Autodesk Fusion 360 part; units mm, degrees
(part 13 of 14)
  arc A3739 (79.673, 23.2351) -> (79.673, 23.4129) centre (79.673, 23.324) ccw
  arc A3740 (71.673, 22.4351) -> (71.673, 22.6129) centre (71.673, 22.524) ccw
  arc A3741 (78.073, 23.4129) -> (78.073, 23.2351) centre (78.073, 23.324) ccw
  arc A3742 (73.273, 22.4351) -> (73.273, 22.6129) centre (73.273, 22.524) ccw
  arc A3743 (73.273, 22.4351) -> (73.273, 22.6129) centre (73.273, 22.524) ccw
  arc A3744 (78.073, 23.4129) -> (78.073, 23.2351) centre (78.073, 23.324) ccw
  arc A3745 (75.673, 23.4129) -> (75.673, 23.2351) centre (75.673, 23.324) ccw
  arc A3746 (74.873, 23.2351) -> (74.873, 23.4129) centre (74.873, 23.324) ccw
  arc A3747 (74.073, 23.4129) -> (74.073, 23.2351) centre (74.073, 23.324) ccw
  arc A3748 (74.073, 23.4129) -> (74.073, 23.2351) centre (74.073, 23.324) ccw
  arc A3749 (74.073, 23.2351) -> (74.073, 23.4129) centre (74.073, 23.324) ccw
  arc A3750 (78.873, 23.4129) -> (78.873, 23.2351) centre (78.873, 23.324) ccw
  arc A3751 (80.473, 23.4129) -> (80.473, 23.2351) centre (80.473, 23.324) ccw
  arc A3752 (78.073, 23.2351) -> (78.073, 23.4129) centre (78.073, 23.324) ccw
  arc A3753 (79.673, 23.4129) -> (79.673, 23.2351) centre (79.673, 23.324) ccw
  arc A3754 (76.473, 23.4129) -> (76.473, 23.2351) centre (76.473, 23.324) ccw
  arc A3755 (74.873, 23.4129) -> (74.873, 23.2351) centre (74.873, 23.324) ccw
  arc A3756 (72.473, 22.4351) -> (72.473, 22.6129) centre (72.473, 22.524) ccw
  arc A3757 (78.073, 23.2351) -> (78.073, 23.4129) centre (78.073, 23.324) ccw
  arc A3758 (76.473, 23.4129) -> (76.473, 23.2351) centre (76.473, 23.324) ccw
  arc A3759 (77.273, 23.4129) -> (77.273, 23.2351) centre (77.273, 23.324) ccw
  arc A3760 (76.473, 23.2351) -> (76.473, 23.4129) centre (76.473, 23.324) ccw
  arc A3761 (78.873, 23.4129) -> (78.873, 23.2351) centre (78.873, 23.324) ccw
  arc A3762 (72.473, 22.6129) -> (72.473, 22.4351) centre (72.473, 22.524) ccw
  arc A3763 (80.473, 23.2351) -> (80.473, 23.4129) centre (80.473, 23.324) ccw
  arc A3764 (71.673, 22.6129) -> (71.673, 22.4351) centre (71.673, 22.524) ccw
  arc A3765 (79.673, 23.2351) -> (79.673, 23.4129) centre (79.673, 23.324) ccw
  arc A3766 (78.873, 23.2351) -> (78.873, 23.4129) centre (78.873, 23.324) ccw
  arc A3767 (79.673, 23.2351) -> (79.673, 23.4129) centre (79.673, 23.324) ccw
  arc A3768 (73.273, 22.6129) -> (73.273, 22.4351) centre (73.273, 22.524) ccw
  arc A3769 (73.273, 23.4129) -> (73.273, 23.2351) centre (73.273, 23.324) ccw
  arc A3770 (71.673, 22.4351) -> (71.673, 22.6129) centre (71.673, 22.524) ccw
  arc A3771 (73.273, 23.2351) -> (73.273, 23.4129) centre (73.273, 23.324) ccw
  arc A3772 (72.473, 22.4351) -> (72.473, 22.6129) centre (72.473, 22.524) ccw
  arc A3773 (71.673, 22.6129) -> (71.673, 22.4351) centre (71.673, 22.524) ccw
  arc A3774 (80.473, 23.2351) -> (80.473, 23.4129) centre (80.473, 23.324) ccw
  arc A3775 (79.673, 23.4129) -> (79.673, 23.2351) centre (79.673, 23.324) ccw
  arc A3776 (78.873, 23.2351) -> (78.873, 23.4129) centre (78.873, 23.324) ccw
  arc A3777 (72.473, 22.6129) -> (72.473, 22.4351) centre (72.473, 22.524) ccw
  arc A3778 (78.073, 23.4129) -> (78.073, 23.2351) centre (78.073, 23.324) ccw
  arc A3779 (76.473, 23.2351) -> (76.473, 23.4129) centre (76.473, 23.324) ccw
  arc A3780 (75.673, 23.2351) -> (75.673, 23.4129) centre (75.673, 23.324) ccw
  arc A3781 (72.473, 22.6129) -> (72.473, 22.4351) centre (72.473, 22.524) ccw
  arc A3782 (78.873, 23.4129) -> (78.873, 23.2351) centre (78.873, 23.324) ccw
  arc A3783 (80.473, 23.2351) -> (80.473, 23.4129) centre (80.473, 23.324) ccw
  arc A3784 (73.273, 23.4129) -> (73.273, 23.2351) centre (73.273, 23.324) ccw
  arc A3785 (76.473, 23.4129) -> (76.473, 23.2351) centre (76.473, 23.324) ccw
  arc A3786 (72.473, 24.0351) -> (72.473, 24.2129) centre (72.473, 24.124) ccw
  arc A3787 (74.073, 24.2129) -> (74.073, 24.0351) centre (74.073, 24.124) ccw
  arc A3788 (76.473, 24.0351) -> (76.473, 24.2129) centre (76.473, 24.124) ccw
  arc A3789 (77.273, 23.4129) -> (77.273, 23.2351) centre (77.273, 23.324) ccw
  arc A3790 (71.673, 23.4129) -> (71.673, 23.2351) centre (71.673, 23.324) ccw
  arc A3791 (77.273, 24.0351) -> (77.273, 24.2129) centre (77.273, 24.124) ccw
  arc A3792 (71.673, 23.4129) -> (71.673, 23.2351) centre (71.673, 23.324) ccw
  arc A3793 (72.473, 23.2351) -> (72.473, 23.4129) centre (72.473, 23.324) ccw
  arc A3794 (78.873, 24.2129) -> (78.873, 24.0351) centre (78.873, 24.124) ccw
  arc A3795 (73.273, 24.2129) -> (73.273, 24.0351) centre (73.273, 24.124) ccw
  arc A3796 (77.273, 23.2351) -> (77.273, 23.4129) centre (77.273, 23.324) ccw
  arc A3797 (78.873, 24.0351) -> (78.873, 24.2129) centre (78.873, 24.124) ccw
  arc A3798 (80.473, 24.2129) -> (80.473, 24.0351) centre (80.473, 24.124) ccw
  arc A3799 (78.073, 24.0351) -> (78.073, 24.2129) centre (78.073, 24.124) ccw
  arc A3800 (78.873, 24.2129) -> (78.873, 24.0351) centre (78.873, 24.124) ccw
  arc A3801 (71.673, 23.4129) -> (71.673, 23.2351) centre (71.673, 23.324) ccw
  arc A3802 (79.673, 24.2129) -> (79.673, 24.0351) centre (79.673, 24.124) ccw
  arc A3803 (74.073, 24.0351) -> (74.073, 24.2129) centre (74.073, 24.124) ccw
  arc A3804 (78.073, 24.2129) -> (78.073, 24.0351) centre (78.073, 24.124) ccw
  arc A3805 (77.273, 24.0351) -> (77.273, 24.2129) centre (77.273, 24.124) ccw
  arc A3806 (78.873, 24.0351) -> (78.873, 24.2129) centre (78.873, 24.124) ccw
  arc A3807 (74.873, 23.4129) -> (74.873, 23.2351) centre (74.873, 23.324) ccw
  arc A3808 (74.073, 23.2351) -> (74.073, 23.4129) centre (74.073, 23.324) ccw
  arc A3809 (79.673, 24.2129) -> (79.673, 24.0351) centre (79.673, 24.124) ccw
  arc A3810 (72.473, 23.4129) -> (72.473, 23.2351) centre (72.473, 23.324) ccw
  arc A3811 (72.473, 23.2351) -> (72.473, 23.4129) centre (72.473, 23.324) ccw
  arc A3812 (74.073, 23.2351) -> (74.073, 23.4129) centre (74.073, 23.324) ccw
  arc A3813 (71.673, 23.2351) -> (71.673, 23.4129) centre (71.673, 23.324) ccw
  arc A3814 (76.473, 24.2129) -> (76.473, 24.0351) centre (76.473, 24.124) ccw
  arc A3815 (73.273, 23.4129) -> (73.273, 23.2351) centre (73.273, 23.324) ccw
  arc A3816 (80.473, 24.2129) -> (80.473, 24.0351) centre (80.473, 24.124) ccw
  arc A3817 (72.473, 23.4129) -> (72.473, 23.2351) centre (72.473, 23.324) ccw
  arc A3818 (71.673, 23.2351) -> (71.673, 23.4129) centre (71.673, 23.324) ccw
  arc A3819 (79.673, 24.0351) -> (79.673, 24.2129) centre (79.673, 24.124) ccw
  arc A3820 (73.273, 24.0351) -> (73.273, 24.2129) centre (73.273, 24.124) ccw
  arc A3821 (74.873, 24.0351) -> (74.873, 24.2129) centre (74.873, 24.124) ccw
  arc A3822 (72.473, 24.0351) -> (72.473, 24.2129) centre (72.473, 24.124) ccw
  arc A3823 (79.673, 24.0351) -> (79.673, 24.2129) centre (79.673, 24.124) ccw
  arc A3824 (78.073, 24.0351) -> (78.073, 24.2129) centre (78.073, 24.124) ccw
  arc A3825 (72.473, 23.4129) -> (72.473, 23.2351) centre (72.473, 23.324) ccw
  arc A3826 (77.273, 24.2129) -> (77.273, 24.0351) centre (77.273, 24.124) ccw
  arc A3827 (75.673, 23.2351) -> (75.673, 23.4129) centre (75.673, 23.324) ccw
  arc A3828 (76.473, 23.2351) -> (76.473, 23.4129) centre (76.473, 23.324) ccw
  arc A3829 (80.473, 24.0351) -> (80.473, 24.2129) centre (80.473, 24.124) ccw
  arc A3830 (73.273, 23.2351) -> (73.273, 23.4129) centre (73.273, 23.324) ccw
  arc A3831 (78.873, 24.0351) -> (78.873, 24.2129) centre (78.873, 24.124) ccw
  arc A3832 (77.273, 24.2129) -> (77.273, 24.0351) centre (77.273, 24.124) ccw
  arc A3833 (77.273, 23.2351) -> (77.273, 23.4129) centre (77.273, 23.324) ccw
  arc A3834 (78.073, 24.2129) -> (78.073, 24.0351) centre (78.073, 24.124) ccw
  arc A3835 (80.473, 24.0351) -> (80.473, 24.2129) centre (80.473, 24.124) ccw
  arc A3836 (80.473, 24.2129) -> (80.473, 24.0351) centre (80.473, 24.124) ccw
  arc A3837 (79.673, 24.2129) -> (79.673, 24.0351) centre (79.673, 24.124) ccw
  arc A3838 (71.673, 23.2351) -> (71.673, 23.4129) centre (71.673, 23.324) ccw
  arc A3839 (79.673, 24.0351) -> (79.673, 24.2129) centre (79.673, 24.124) ccw
  arc A3840 (78.073, 24.2129) -> (78.073, 24.0351) centre (78.073, 24.124) ccw
  arc A3841 (78.873, 24.2129) -> (78.873, 24.0351) centre (78.873, 24.124) ccw
  arc A3842 (77.273, 24.2129) -> (77.273, 24.0351) centre (77.273, 24.124) ccw
  arc A3843 (75.673, 23.4129) -> (75.673, 23.2351) centre (75.673, 23.324) ccw
  arc A3844 (72.473, 23.2351) -> (72.473, 23.4129) centre (72.473, 23.324) ccw
  arc A3845 (74.073, 24.2129) -> (74.073, 24.0351) centre (74.073, 24.124) ccw
  arc A3846 (74.073, 24.0351) -> (74.073, 24.2129) centre (74.073, 24.124) ccw
  arc A3847 (73.273, 24.2129) -> (73.273, 24.0351) centre (73.273, 24.124) ccw
  arc A3848 (78.073, 24.0351) -> (78.073, 24.2129) centre (78.073, 24.124) ccw
  arc A3849 (80.473, 24.0351) -> (80.473, 24.2129) centre (80.473, 24.124) ccw
  arc A3850 (80.473, 24.8351) -> (80.473, 25.0129) centre (80.473, 24.924) ccw
  arc A3851 (78.873, 25.0129) -> (78.873, 24.8351) centre (78.873, 24.924) ccw
  arc A3852 (77.273, 25.0129) -> (77.273, 24.8351) centre (77.273, 24.924) ccw
  arc A3853 (78.073, 24.8351) -> (78.073, 25.0129) centre (78.073, 24.924) ccw
  arc A3854 (72.473, 24.2129) -> (72.473, 24.0351) centre (72.473, 24.124) ccw
  arc A3855 (79.673, 25.0129) -> (79.673, 24.8351) centre (79.673, 24.924) ccw
  arc A3856 (74.873, 24.0351) -> (74.873, 24.2129) centre (74.873, 24.124) ccw
  arc A3857 (78.873, 24.8351) -> (78.873, 25.0129) centre (78.873, 24.924) ccw
  arc A3858 (80.473, 24.8351) -> (80.473, 25.0129) centre (80.473, 24.924) ccw
  arc A3859 (75.673, 24.0351) -> (75.673, 24.2129) centre (75.673, 24.124) ccw
  arc A3860 (73.273, 24.0351) -> (73.273, 24.2129) centre (73.273, 24.124) ccw
  arc A3861 (71.673, 24.2129) -> (71.673, 24.0351) centre (71.673, 24.124) ccw
  arc A3862 (75.673, 24.2129) -> (75.673, 24.0351) centre (75.673, 24.124) ccw
  arc A3863 (79.673, 25.0129) -> (79.673, 24.8351) centre (79.673, 24.924) ccw
  arc A3864 (78.073, 25.0129) -> (78.073, 24.8351) centre (78.073, 24.924) ccw
  arc A3865 (77.273, 24.0351) -> (77.273, 24.2129) centre (77.273, 24.124) ccw
  arc A3866 (73.273, 24.2129) -> (73.273, 24.0351) centre (73.273, 24.124) ccw
  arc A3867 (78.873, 24.8351) -> (78.873, 25.0129) centre (78.873, 24.924) ccw
  arc A3868 (80.473, 25.0129) -> (80.473, 24.8351) centre (80.473, 24.924) ccw
  arc A3869 (77.273, 24.8351) -> (77.273, 25.0129) centre (77.273, 24.924) ccw
  arc A3870 (78.073, 24.8351) -> (78.073, 25.0129) centre (78.073, 24.924) ccw
  arc A3871 (75.673, 24.0351) -> (75.673, 24.2129) centre (75.673, 24.124) ccw
  arc A3872 (78.873, 25.0129) -> (78.873, 24.8351) centre (78.873, 24.924) ccw
  arc A3873 (78.073, 25.0129) -> (78.073, 24.8351) centre (78.073, 24.924) ccw
  arc A3874 (78.073, 25.0129) -> (78.073, 24.8351) centre (78.073, 24.924) ccw
  arc A3875 (80.473, 25.0129) -> (80.473, 24.8351) centre (80.473, 24.924) ccw
  arc A3876 (53.735, 36.8717) -> (53.735, 37.1384) centre (53.735, 37.005) ccw
  arc A3877 (57.735, 36.8717) -> (57.735, 37.1384) centre (57.735, 37.005) ccw
  arc A3878 (71.673, 24.0351) -> (71.673, 24.2129) centre (71.673, 24.124) ccw
  arc A3879 (79.673, 24.8351) -> (79.673, 25.0129) centre (79.673, 24.924) ccw
  arc A3880 (57.735, 36.8717) -> (57.735, 37.1384) centre (57.735, 37.005) ccw
  arc A3881 (54.735, 36.8717) -> (54.735, 37.1384) centre (54.735, 37.005) ccw
  arc A3882 (54.735, 37.1384) -> (54.735, 36.8717) centre (54.735, 37.005) ccw
  arc A3883 (53.735, 37.1384) -> (53.735, 36.8717) centre (53.735, 37.005) ccw
  arc A3884 (55.735, 36.8717) -> (55.735, 37.1384) centre (55.735, 37.005) ccw
  arc A3885 (75.673, 24.2129) -> (75.673, 24.0351) centre (75.673, 24.124) ccw
  arc A3886 (79.673, 24.8351) -> (79.673, 25.0129) centre (79.673, 24.924) ccw
  arc A3887 (72.473, 24.2129) -> (72.473, 24.0351) centre (72.473, 24.124) ccw
  arc A3888 (73.273, 24.0351) -> (73.273, 24.2129) centre (73.273, 24.124) ccw
  arc A3889 (72.473, 24.0351) -> (72.473, 24.2129) centre (72.473, 24.124) ccw
  arc A3890 (75.673, 24.0351) -> (75.673, 24.2129) centre (75.673, 24.124) ccw
  arc A3891 (74.873, 24.2129) -> (74.873, 24.0351) centre (74.873, 24.124) ccw
  arc A3892 (76.473, 24.2129) -> (76.473, 24.0351) centre (76.473, 24.124) ccw
  arc A3893 (76.473, 24.0351) -> (76.473, 24.2129) centre (76.473, 24.124) ccw
  arc A3894 (74.873, 24.0351) -> (74.873, 24.2129) centre (74.873, 24.124) ccw
  arc A3895 (72.473, 24.2129) -> (72.473, 24.0351) centre (72.473, 24.124) ccw
  arc A3896 (76.473, 24.2129) -> (76.473, 24.0351) centre (76.473, 24.124) ccw
  arc A3897 (74.873, 24.2129) -> (74.873, 24.0351) centre (74.873, 24.124) ccw
  arc A3898 (74.073, 24.2129) -> (74.073, 24.0351) centre (74.073, 24.124) ccw
  arc A3899 (74.873, 24.2129) -> (74.873, 24.0351) centre (74.873, 24.124) ccw
  arc A3900 (78.073, 24.8351) -> (78.073, 25.0129) centre (78.073, 24.924) ccw
  arc A3901 (74.073, 24.0351) -> (74.073, 24.2129) centre (74.073, 24.124) ccw
  arc A3902 (76.473, 24.0351) -> (76.473, 24.2129) centre (76.473, 24.124) ccw
  arc A3903 (71.673, 24.2129) -> (71.673, 24.0351) centre (71.673, 24.124) ccw
  arc A3904 (71.673, 24.2129) -> (71.673, 24.0351) centre (71.673, 24.124) ccw
  arc A3905 (79.673, 24.8351) -> (79.673, 25.0129) centre (79.673, 24.924) ccw
  arc A3906 (78.873, 25.0129) -> (78.873, 24.8351) centre (78.873, 24.924) ccw
  arc A3907 (79.673, 25.0129) -> (79.673, 24.8351) centre (79.673, 24.924) ccw
  arc A3908 (71.673, 24.0351) -> (71.673, 24.2129) centre (71.673, 24.124) ccw
  arc A3909 (78.873, 24.8351) -> (78.873, 25.0129) centre (78.873, 24.924) ccw
  arc A3910 (80.473, 25.0129) -> (80.473, 24.8351) centre (80.473, 24.924) ccw
  arc A3911 (80.473, 24.8351) -> (80.473, 25.0129) centre (80.473, 24.924) ccw
  arc A3912 (75.673, 24.2129) -> (75.673, 24.0351) centre (75.673, 24.124) ccw
  arc A3913 (71.673, 24.0351) -> (71.673, 24.2129) centre (71.673, 24.124) ccw
  arc A3914 (54.735, 37.1384) -> (54.735, 36.8717) centre (54.735, 37.005) ccw
  arc A3915 (74.873, 25.0129) -> (74.873, 24.8351) centre (74.873, 24.924) ccw
  arc A3916 (74.873, 24.8351) -> (74.873, 25.0129) centre (74.873, 24.924) ccw
  arc A3917 (73.273, 24.8351) -> (73.273, 25.0129) centre (73.273, 24.924) ccw
  arc A3918 (74.073, 24.8351) -> (74.073, 25.0129) centre (74.073, 24.924) ccw
  arc A3919 (72.473, 25.0129) -> (72.473, 24.8351) centre (72.473, 24.924) ccw
  arc A3920 (74.873, 25.0129) -> (74.873, 24.8351) centre (74.873, 24.924) ccw
  arc A3921 (76.473, 25.0129) -> (76.473, 24.8351) centre (76.473, 24.924) ccw
  arc A3922 (56.735, 37.1384) -> (56.735, 36.8717) centre (56.735, 37.005) ccw
  arc A3923 (75.673, 25.0129) -> (75.673, 24.8351) centre (75.673, 24.924) ccw
  arc A3924 (75.673, 24.8351) -> (75.673, 25.0129) centre (75.673, 24.924) ccw
  arc A3925 (56.735, 36.8717) -> (56.735, 37.1384) centre (56.735, 37.005) ccw
  arc A3926 (76.473, 25.0129) -> (76.473, 24.8351) centre (76.473, 24.924) ccw
  arc A3927 (55.735, 37.1384) -> (55.735, 36.8717) centre (55.735, 37.005) ccw
  arc A3928 (55.735, 36.8717) -> (55.735, 37.1384) centre (55.735, 37.005) ccw
  arc A3929 (75.673, 24.8351) -> (75.673, 25.0129) centre (75.673, 24.924) ccw
  arc A3930 (73.273, 25.0129) -> (73.273, 24.8351) centre (73.273, 24.924) ccw
  arc A3931 (72.473, 24.8351) -> (72.473, 25.0129) centre (72.473, 24.924) ccw
  arc A3932 (78.873, 25.6351) -> (78.873, 25.8129) centre (78.873, 25.724) ccw
  arc A3933 (76.473, 25.0129) -> (76.473, 24.8351) centre (76.473, 24.924) ccw
  arc A3934 (53.735, 36.8717) -> (53.735, 37.1384) centre (53.735, 37.005) ccw
  arc A3935 (57.735, 36.8717) -> (57.735, 37.1384) centre (57.735, 37.005) ccw
  arc A3936 (55.735, 36.8717) -> (55.735, 37.1384) centre (55.735, 37.005) ccw
  arc A3937 (78.073, 25.6351) -> (78.073, 25.8129) centre (78.073, 25.724) ccw
  arc A3938 (77.273, 25.6351) -> (77.273, 25.8129) centre (77.273, 25.724) ccw
  arc A3939 (79.673, 25.8129) -> (79.673, 25.6351) centre (79.673, 25.724) ccw
  arc A3940 (75.673, 24.8351) -> (75.673, 25.0129) centre (75.673, 24.924) ccw
  arc A3941 (78.873, 25.6351) -> (78.873, 25.8129) centre (78.873, 25.724) ccw
  arc A3942 (75.673, 25.0129) -> (75.673, 24.8351) centre (75.673, 24.924) ccw
  arc A3943 (75.673, 25.0129) -> (75.673, 24.8351) centre (75.673, 24.924) ccw
  arc A3944 (56.735, 37.1384) -> (56.735, 36.8717) centre (56.735, 37.005) ccw
  arc A3945 (55.735, 37.1384) -> (55.735, 36.8717) centre (55.735, 37.005) ccw
  arc A3946 (74.073, 25.0129) -> (74.073, 24.8351) centre (74.073, 24.924) ccw
  arc A3947 (73.273, 25.0129) -> (73.273, 24.8351) centre (73.273, 24.924) ccw
  arc A3948 (53.735, 36.8717) -> (53.735, 37.1384) centre (53.735, 37.005) ccw
  arc A3949 (74.873, 25.0129) -> (74.873, 24.8351) centre (74.873, 24.924) ccw
  arc A3950 (54.735, 36.8717) -> (54.735, 37.1384) centre (54.735, 37.005) ccw
  arc A3951 (54.735, 37.1384) -> (54.735, 36.8717) centre (54.735, 37.005) ccw
  arc A3952 (72.473, 24.8351) -> (72.473, 25.0129) centre (72.473, 24.924) ccw
  arc A3953 (53.735, 37.1384) -> (53.735, 36.8717) centre (53.735, 37.005) ccw
  arc A3954 (73.273, 25.0129) -> (73.273, 24.8351) centre (73.273, 24.924) ccw
  arc A3955 (72.473, 24.8351) -> (72.473, 25.0129) centre (72.473, 24.924) ccw
  arc A3956 (56.735, 36.8717) -> (56.735, 37.1384) centre (56.735, 37.005) ccw
  arc A3957 (57.735, 37.1384) -> (57.735, 36.8717) centre (57.735, 37.005) ccw
  arc A3958 (76.473, 24.8351) -> (76.473, 25.0129) centre (76.473, 24.924) ccw
  arc A3959 (76.473, 24.8351) -> (76.473, 25.0129) centre (76.473, 24.924) ccw
  arc A3960 (55.735, 37.1384) -> (55.735, 36.8717) centre (55.735, 37.005) ccw
  arc A3961 (74.073, 25.0129) -> (74.073, 24.8351) centre (74.073, 24.924) ccw
  arc A3962 (74.073, 24.8351) -> (74.073, 25.0129) centre (74.073, 24.924) ccw
  arc A3963 (56.735, 37.1384) -> (56.735, 36.8717) centre (56.735, 37.005) ccw
  arc A3964 (74.073, 24.8351) -> (74.073, 25.0129) centre (74.073, 24.924) ccw
  arc A3965 (57.735, 37.1384) -> (57.735, 36.8717) centre (57.735, 37.005) ccw
  arc A3966 (72.473, 25.0129) -> (72.473, 24.8351) centre (72.473, 24.924) ccw
  arc A3967 (76.473, 24.8351) -> (76.473, 25.0129) centre (76.473, 24.924) ccw
  arc A3968 (56.735, 36.8717) -> (56.735, 37.1384) centre (56.735, 37.005) ccw
  arc A3969 (74.873, 24.8351) -> (74.873, 25.0129) centre (74.873, 24.924) ccw
  arc A3970 (72.473, 25.0129) -> (72.473, 24.8351) centre (72.473, 24.924) ccw
  arc A3971 (57.735, 37.1384) -> (57.735, 36.8717) centre (57.735, 37.005) ccw
  arc A3972 (53.735, 37.1384) -> (53.735, 36.8717) centre (53.735, 37.005) ccw
  arc A3973 (74.873, 24.8351) -> (74.873, 25.0129) centre (74.873, 24.924) ccw
  arc A3974 (73.273, 24.8351) -> (73.273, 25.0129) centre (73.273, 24.924) ccw
  arc A3975 (74.073, 25.0129) -> (74.073, 24.8351) centre (74.073, 24.924) ccw
  arc A3976 (54.735, 36.8717) -> (54.735, 37.1384) centre (54.735, 37.005) ccw
  arc A3977 (73.273, 24.8351) -> (73.273, 25.0129) centre (73.273, 24.924) ccw
  arc A3978 (76.473, 25.6351) -> (76.473, 25.8129) centre (76.473, 25.724) ccw
  arc A3979 (74.873, 25.8129) -> (74.873, 25.6351) centre (74.873, 25.724) ccw
  arc A3980 (71.673, 25.0129) -> (71.673, 24.8351) centre (71.673, 24.924) ccw
  arc A3981 (74.873, 25.8129) -> (74.873, 25.6351) centre (74.873, 25.724) ccw
  arc A3982 (73.273, 25.6351) -> (73.273, 25.8129) centre (73.273, 25.724) ccw
  arc A3983 (79.673, 25.8129) -> (79.673, 25.6351) centre (79.673, 25.724) ccw
  arc A3984 (80.473, 25.6351) -> (80.473, 25.8129) centre (80.473, 25.724) ccw
  arc A3985 (79.673, 25.8129) -> (79.673, 25.6351) centre (79.673, 25.724) ccw
  arc A3986 (71.673, 25.6351) -> (71.673, 25.8129) centre (71.673, 25.724) ccw
  arc A3987 (74.873, 25.6351) -> (74.873, 25.8129) centre (74.873, 25.724) ccw
  arc A3988 (76.473, 25.6351) -> (76.473, 25.8129) centre (76.473, 25.724) ccw
  arc A3989 (72.473, 25.8129) -> (72.473, 25.6351) centre (72.473, 25.724) ccw
  arc A3990 (72.473, 25.6351) -> (72.473, 25.8129) centre (72.473, 25.724) ccw
  arc A3991 (72.473, 25.6351) -> (72.473, 25.8129) centre (72.473, 25.724) ccw
  arc A3992 (78.073, 25.8129) -> (78.073, 25.6351) centre (78.073, 25.724) ccw
  arc A3993 (78.873, 25.8129) -> (78.873, 25.6351) centre (78.873, 25.724) ccw
  arc A3994 (76.473, 25.6351) -> (76.473, 25.8129) centre (76.473, 25.724) ccw
  arc A3995 (79.673, 25.6351) -> (79.673, 25.8129) centre (79.673, 25.724) ccw
  arc A3996 (77.273, 25.8129) -> (77.273, 25.6351) centre (77.273, 25.724) ccw
  arc A3997 (71.673, 25.0129) -> (71.673, 24.8351) centre (71.673, 24.924) ccw
  arc A3998 (73.273, 25.8129) -> (73.273, 25.6351) centre (73.273, 25.724) ccw
  arc A3999 (80.473, 25.8129) -> (80.473, 25.6351) centre (80.473, 25.724) ccw
  arc A4000 (77.273, 25.6351) -> (77.273, 25.8129) centre (77.273, 25.724) ccw
  arc A4001 (78.873, 25.8129) -> (78.873, 25.6351) centre (78.873, 25.724) ccw
  arc A4002 (76.473, 25.8129) -> (76.473, 25.6351) centre (76.473, 25.724) ccw
  arc A4003 (80.473, 25.8129) -> (80.473, 25.6351) centre (80.473, 25.724) ccw
  arc A4004 (74.073, 25.6351) -> (74.073, 25.8129) centre (74.073, 25.724) ccw
  arc A4005 (73.273, 25.6351) -> (73.273, 25.8129) centre (73.273, 25.724) ccw
  arc A4006 (77.273, 25.8129) -> (77.273, 25.6351) centre (77.273, 25.724) ccw
  arc A4007 (75.673, 25.6351) -> (75.673, 25.8129) centre (75.673, 25.724) ccw
  arc A4008 (74.073, 25.6351) -> (74.073, 25.8129) centre (74.073, 25.724) ccw
  arc A4009 (73.273, 25.8129) -> (73.273, 25.6351) centre (73.273, 25.724) ccw
  arc A4010 (74.073, 25.8129) -> (74.073, 25.6351) centre (74.073, 25.724) ccw
  arc A4011 (75.673, 25.6351) -> (75.673, 25.8129) centre (75.673, 25.724) ccw
  arc A4012 (71.673, 25.8129) -> (71.673, 25.6351) centre (71.673, 25.724) ccw
  arc A4013 (71.673, 25.0129) -> (71.673, 24.8351) centre (71.673, 24.924) ccw
  arc A4014 (80.473, 25.6351) -> (80.473, 25.8129) centre (80.473, 25.724) ccw
  arc A4015 (77.273, 25.8129) -> (77.273, 25.6351) centre (77.273, 25.724) ccw
  arc A4016 (76.473, 25.8129) -> (76.473, 25.6351) centre (76.473, 25.724) ccw
  arc A4017 (78.073, 25.8129) -> (78.073, 25.6351) centre (78.073, 25.724) ccw
  arc A4018 (80.473, 25.8129) -> (80.473, 25.6351) centre (80.473, 25.724) ccw
  arc A4019 (78.073, 25.6351) -> (78.073, 25.8129) centre (78.073, 25.724) ccw
  arc A4020 (79.673, 25.6351) -> (79.673, 25.8129) centre (79.673, 25.724) ccw
  arc A4021 (71.673, 24.8351) -> (71.673, 25.0129) centre (71.673, 24.924) ccw
  arc A4022 (80.473, 25.6351) -> (80.473, 25.8129) centre (80.473, 25.724) ccw
  arc A4023 (78.873, 25.8129) -> (78.873, 25.6351) centre (78.873, 25.724) ccw
  arc A4024 (77.273, 25.6351) -> (77.273, 25.8129) centre (77.273, 25.724) ccw
  arc A4025 (78.873, 25.6351) -> (78.873, 25.8129) centre (78.873, 25.724) ccw
  arc A4026 (71.673, 24.8351) -> (71.673, 25.0129) centre (71.673, 24.924) ccw
  arc A4027 (78.073, 25.8129) -> (78.073, 25.6351) centre (78.073, 25.724) ccw
  arc A4028 (71.673, 24.8351) -> (71.673, 25.0129) centre (71.673, 24.924) ccw
  arc A4029 (78.073, 25.6351) -> (78.073, 25.8129) centre (78.073, 25.724) ccw
  arc A4030 (79.673, 25.6351) -> (79.673, 25.8129) centre (79.673, 25.724) ccw
  arc A4031 (76.473, 25.8129) -> (76.473, 25.6351) centre (76.473, 25.724) ccw
  arc A4032 (75.673, 25.6351) -> (75.673, 25.8129) centre (75.673, 25.724) ccw
  arc A4033 (72.473, 25.6351) -> (72.473, 25.8129) centre (72.473, 25.724) ccw
  arc A4034 (71.673, 25.8129) -> (71.673, 25.6351) centre (71.673, 25.724) ccw
  arc A4035 (75.673, 25.8129) -> (75.673, 25.6351) centre (75.673, 25.724) ccw
  arc A4036 (73.273, 25.6351) -> (73.273, 25.8129) centre (73.273, 25.724) ccw
  arc A4037 (74.873, 25.6351) -> (74.873, 25.8129) centre (74.873, 25.724) ccw
  arc A4038 (74.073, 25.6351) -> (74.073, 25.8129) centre (74.073, 25.724) ccw
  arc A4039 (72.473, 25.8129) -> (72.473, 25.6351) centre (72.473, 25.724) ccw
  arc A4040 (72.473, 25.8129) -> (72.473, 25.6351) centre (72.473, 25.724) ccw
  arc A4041 (75.673, 25.8129) -> (75.673, 25.6351) centre (75.673, 25.724) ccw
  arc A4042 (71.673, 26.4351) -> (71.673, 26.6129) centre (71.673, 26.524) ccw
  arc A4043 (71.673, 26.4351) -> (71.673, 26.6129) centre (71.673, 26.524) ccw
  arc A4044 (76.473, 26.6129) -> (76.473, 26.4351) centre (76.473, 26.524) ccw
  arc A4045 (73.273, 26.6129) -> (73.273, 26.4351) centre (73.273, 26.524) ccw
  arc A4046 (74.873, 25.8129) -> (74.873, 25.6351) centre (74.873, 25.724) ccw
  arc A4047 (78.073, 26.4351) -> (78.073, 26.6129) centre (78.073, 26.524) ccw
  arc A4048 (78.873, 26.4351) -> (78.873, 26.6129) centre (78.873, 26.524) ccw
  arc A4049 (73.273, 25.8129) -> (73.273, 25.6351) centre (73.273, 25.724) ccw
  arc A4050 (79.673, 26.6129) -> (79.673, 26.4351) centre (79.673, 26.524) ccw
  arc A4051 (78.873, 26.4351) -> (78.873, 26.6129) centre (78.873, 26.524) ccw
  arc A4052 (76.473, 26.6129) -> (76.473, 26.4351) centre (76.473, 26.524) ccw
  arc A4053 (73.273, 26.6129) -> (73.273, 26.4351) centre (73.273, 26.524) ccw
  arc A4054 (80.473, 26.6129) -> (80.473, 26.4351) centre (80.473, 26.524) ccw
  arc A4055 (71.673, 25.6351) -> (71.673, 25.8129) centre (71.673, 25.724) ccw
  arc A4056 (76.473, 26.4351) -> (76.473, 26.6129) centre (76.473, 26.524) ccw
  arc A4057 (77.273, 26.4351) -> (77.273, 26.6129) centre (77.273, 26.524) ccw
  arc A4058 (80.473, 26.4351) -> (80.473, 26.6129) centre (80.473, 26.524) ccw
  arc A4059 (80.473, 26.6129) -> (80.473, 26.4351) centre (80.473, 26.524) ccw
  arc A4060 (80.473, 26.4351) -> (80.473, 26.6129) centre (80.473, 26.524) ccw
  arc A4061 (77.273, 26.6129) -> (77.273, 26.4351) centre (77.273, 26.524) ccw
  arc A4062 (73.273, 26.4351) -> (73.273, 26.6129) centre (73.273, 26.524) ccw
  arc A4063 (80.473, 26.6129) -> (80.473, 26.4351) centre (80.473, 26.524) ccw
  arc A4064 (78.073, 26.4351) -> (78.073, 26.6129) centre (78.073, 26.524) ccw
  arc A4065 (72.473, 26.4351) -> (72.473, 26.6129) centre (72.473, 26.524) ccw
  arc A4066 (75.673, 26.6129) -> (75.673, 26.4351) centre (75.673, 26.524) ccw
  arc A4067 (74.873, 26.6129) -> (74.873, 26.4351) centre (74.873, 26.524) ccw
  arc A4068 (74.873, 26.6129) -> (74.873, 26.4351) centre (74.873, 26.524) ccw
  arc A4069 (71.673, 26.6129) -> (71.673, 26.4351) centre (71.673, 26.524) ccw
  arc A4070 (77.273, 26.6129) -> (77.273, 26.4351) centre (77.273, 26.524) ccw
  arc A4071 (71.673, 26.4351) -> (71.673, 26.6129) centre (71.673, 26.524) ccw
  arc A4072 (74.873, 25.6351) -> (74.873, 25.8129) centre (74.873, 25.724) ccw
  arc A4073 (71.673, 26.6129) -> (71.673, 26.4351) centre (71.673, 26.524) ccw
  arc A4074 (80.473, 27.4129) -> (80.473, 27.2351) centre (80.473, 27.324) ccw
  arc A4075 (71.673, 26.6129) -> (71.673, 26.4351) centre (71.673, 26.524) ccw
  arc A4076 (72.473, 26.6129) -> (72.473, 26.4351) centre (72.473, 26.524) ccw
  arc A4077 (79.673, 26.4351) -> (79.673, 26.6129) centre (79.673, 26.524) ccw
  arc A4078 (76.473, 26.6129) -> (76.473, 26.4351) centre (76.473, 26.524) ccw
  arc A4079 (74.073, 25.8129) -> (74.073, 25.6351) centre (74.073, 25.724) ccw
  arc A4080 (71.673, 25.8129) -> (71.673, 25.6351) centre (71.673, 25.724) ccw
  arc A4081 (78.873, 26.6129) -> (78.873, 26.4351) centre (78.873, 26.524) ccw
  arc A4082 (78.073, 26.6129) -> (78.073, 26.4351) centre (78.073, 26.524) ccw
  arc A4083 (79.673, 26.6129) -> (79.673, 26.4351) centre (79.673, 26.524) ccw
  arc A4084 (77.273, 26.6129) -> (77.273, 26.4351) centre (77.273, 26.524) ccw
  arc A4085 (80.473, 26.4351) -> (80.473, 26.6129) centre (80.473, 26.524) ccw
  arc A4086 (78.873, 26.6129) -> (78.873, 26.4351) centre (78.873, 26.524) ccw
  arc A4087 (78.073, 26.4351) -> (78.073, 26.6129) centre (78.073, 26.524) ccw
  arc A4088 (79.673, 26.4351) -> (79.673, 26.6129) centre (79.673, 26.524) ccw
  arc A4089 (78.873, 26.4351) -> (78.873, 26.6129) centre (78.873, 26.524) ccw
  arc A4090 (71.673, 25.6351) -> (71.673, 25.8129) centre (71.673, 25.724) ccw
  arc A4091 (79.673, 26.6129) -> (79.673, 26.4351) centre (79.673, 26.524) ccw
  arc A4092 (76.473, 26.4351) -> (76.473, 26.6129) centre (76.473, 26.524) ccw
  arc A4093 (75.673, 25.8129) -> (75.673, 25.6351) centre (75.673, 25.724) ccw
  arc A4094 (79.673, 26.4351) -> (79.673, 26.6129) centre (79.673, 26.524) ccw
  arc A4095 (78.873, 26.6129) -> (78.873, 26.4351) centre (78.873, 26.524) ccw
  arc A4096 (78.073, 26.6129) -> (78.073, 26.4351) centre (78.073, 26.524) ccw
  arc A4097 (77.273, 26.4351) -> (77.273, 26.6129) centre (77.273, 26.524) ccw
  arc A4098 (77.273, 26.4351) -> (77.273, 26.6129) centre (77.273, 26.524) ccw
  arc A4099 (76.473, 26.4351) -> (76.473, 26.6129) centre (76.473, 26.524) ccw
  arc A4100 (74.073, 25.8129) -> (74.073, 25.6351) centre (74.073, 25.724) ccw
  arc A4101 (78.073, 26.6129) -> (78.073, 26.4351) centre (78.073, 26.524) ccw
  arc A4102 (75.673, 26.6129) -> (75.673, 26.4351) centre (75.673, 26.524) ccw
  arc A4103 (74.073, 26.4351) -> (74.073, 26.6129) centre (74.073, 26.524) ccw
  arc A4104 (72.473, 26.6129) -> (72.473, 26.4351) centre (72.473, 26.524) ccw
  arc A4105 (74.873, 26.4351) -> (74.873, 26.6129) centre (74.873, 26.524) ccw
  arc A4106 (75.673, 27.4129) -> (75.673, 27.2351) centre (75.673, 27.324) ccw
  arc A4107 (78.873, 27.4129) -> (78.873, 27.2351) centre (78.873, 27.324) ccw
  arc A4108 (74.073, 26.6129) -> (74.073, 26.4351) centre (74.073, 26.524) ccw
  arc A4109 (76.473, 27.2351) -> (76.473, 27.4129) centre (76.473, 27.324) ccw
  arc A4110 (80.473, 27.2351) -> (80.473, 27.4129) centre (80.473, 27.324) ccw
  arc A4111 (75.673, 27.2351) -> (75.673, 27.4129) centre (75.673, 27.324) ccw
  arc A4112 (77.273, 27.2351) -> (77.273, 27.4129) centre (77.273, 27.324) ccw
  arc A4113 (73.273, 26.6129) -> (73.273, 26.4351) centre (73.273, 26.524) ccw
  arc A4114 (78.073, 27.2351) -> (78.073, 27.4129) centre (78.073, 27.324) ccw
  arc A4115 (77.273, 27.4129) -> (77.273, 27.2351) centre (77.273, 27.324) ccw
  arc A4116 (75.673, 27.4129) -> (75.673, 27.2351) centre (75.673, 27.324) ccw
  arc A4117 (73.273, 26.4351) -> (73.273, 26.6129) centre (73.273, 26.524) ccw
  arc A4118 (79.673, 27.2351) -> (79.673, 27.4129) centre (79.673, 27.324) ccw
  arc A4119 (75.673, 26.6129) -> (75.673, 26.4351) centre (75.673, 26.524) ccw
  arc A4120 (75.673, 27.2351) -> (75.673, 27.4129) centre (75.673, 27.324) ccw
  arc A4121 (80.473, 27.2351) -> (80.473, 27.4129) centre (80.473, 27.324) ccw
  arc A4122 (79.673, 27.4129) -> (79.673, 27.2351) centre (79.673, 27.324) ccw
  arc A4123 (78.873, 27.2351) -> (78.873, 27.4129) centre (78.873, 27.324) ccw
  arc A4124 (78.873, 27.2351) -> (78.873, 27.4129) centre (78.873, 27.324) ccw
  arc A4125 (78.873, 27.2351) -> (78.873, 27.4129) centre (78.873, 27.324) ccw
  arc A4126 (72.473, 26.4351) -> (72.473, 26.6129) centre (72.473, 26.524) ccw
  arc A4127 (74.073, 27.4129) -> (74.073, 27.2351) centre (74.073, 27.324) ccw
  arc A4128 (80.473, 28.2129) -> (80.473, 28.0351) centre (80.473, 28.124) ccw
  arc A4129 (78.073, 27.4129) -> (78.073, 27.2351) centre (78.073, 27.324) ccw
  arc A4130 (80.473, 28.0351) -> (80.473, 28.2129) centre (80.473, 28.124) ccw
  arc A4131 (73.273, 27.4129) -> (73.273, 27.2351) centre (73.273, 27.324) ccw
  arc A4132 (75.673, 26.4351) -> (75.673, 26.6129) centre (75.673, 26.524) ccw
  arc A4133 (73.273, 27.2351) -> (73.273, 27.4129) centre (73.273, 27.324) ccw
  arc A4134 (77.273, 27.4129) -> (77.273, 27.2351) centre (77.273, 27.324) ccw
  arc A4135 (80.473, 27.2351) -> (80.473, 27.4129) centre (80.473, 27.324) ccw
  arc A4136 (75.673, 26.4351) -> (75.673, 26.6129) centre (75.673, 26.524) ccw
  arc A4137 (74.073, 26.4351) -> (74.073, 26.6129) centre (74.073, 26.524) ccw
  arc A4138 (74.073, 26.6129) -> (74.073, 26.4351) centre (74.073, 26.524) ccw
  arc A4139 (76.473, 27.2351) -> (76.473, 27.4129) centre (76.473, 27.324) ccw
  arc A4140 (79.673, 27.2351) -> (79.673, 27.4129) centre (79.673, 27.324) ccw
  arc A4141 (77.273, 27.2351) -> (77.273, 27.4129) centre (77.273, 27.324) ccw
  arc A4142 (76.473, 27.4129) -> (76.473, 27.2351) centre (76.473, 27.324) ccw
  arc A4143 (73.273, 26.4351) -> (73.273, 26.6129) centre (73.273, 26.524) ccw
  arc A4144 (78.873, 27.4129) -> (78.873, 27.2351) centre (78.873, 27.324) ccw
  arc A4145 (75.673, 26.4351) -> (75.673, 26.6129) centre (75.673, 26.524) ccw
  arc A4146 (78.073, 27.2351) -> (78.073, 27.4129) centre (78.073, 27.324) ccw
  arc A4147 (75.673, 27.4129) -> (75.673, 27.2351) centre (75.673, 27.324) ccw
  arc A4148 (74.873, 26.4351) -> (74.873, 26.6129) centre (74.873, 26.524) ccw
  arc A4149 (76.473, 27.4129) -> (76.473, 27.2351) centre (76.473, 27.324) ccw
  arc A4150 (79.673, 27.4129) -> (79.673, 27.2351) centre (79.673, 27.324) ccw
  arc A4151 (77.273, 27.4129) -> (77.273, 27.2351) centre (77.273, 27.324) ccw
  arc A4152 (75.673, 27.2351) -> (75.673, 27.4129) centre (75.673, 27.324) ccw
  arc A4153 (78.873, 27.4129) -> (78.873, 27.2351) centre (78.873, 27.324) ccw
  arc A4154 (78.073, 27.4129) -> (78.073, 27.2351) centre (78.073, 27.324) ccw
  arc A4155 (72.473, 26.6129) -> (72.473, 26.4351) centre (72.473, 26.524) ccw
  arc A4156 (80.473, 27.4129) -> (80.473, 27.2351) centre (80.473, 27.324) ccw
  arc A4157 (79.673, 27.4129) -> (79.673, 27.2351) centre (79.673, 27.324) ccw
  arc A4158 (77.273, 27.2351) -> (77.273, 27.4129) centre (77.273, 27.324) ccw
  arc A4159 (79.673, 27.2351) -> (79.673, 27.4129) centre (79.673, 27.324) ccw
  arc A4160 (72.473, 26.4351) -> (72.473, 26.6129) centre (72.473, 26.524) ccw
  arc A4161 (74.073, 26.4351) -> (74.073, 26.6129) centre (74.073, 26.524) ccw
  arc A4162 (78.073, 27.2351) -> (78.073, 27.4129) centre (78.073, 27.324) ccw
  arc A4163 (74.073, 26.6129) -> (74.073, 26.4351) centre (74.073, 26.524) ccw
  arc A4164 (74.873, 26.6129) -> (74.873, 26.4351) centre (74.873, 26.524) ccw
  arc A4165 (74.873, 26.4351) -> (74.873, 26.6129) centre (74.873, 26.524) ccw
  arc A4166 (80.473, 27.4129) -> (80.473, 27.2351) centre (80.473, 27.324) ccw
  arc A4167 (76.473, 27.4129) -> (76.473, 27.2351) centre (76.473, 27.324) ccw
  arc A4168 (76.473, 27.2351) -> (76.473, 27.4129) centre (76.473, 27.324) ccw
  arc A4169 (78.073, 27.4129) -> (78.073, 27.2351) centre (78.073, 27.324) ccw
  line L6141 (78.656, 35.418) -> (79.456, 35.418)
  line L6142 (75.227, 36.718) -> (76.027, 36.718)
  arc A4170 (71.673, 27.4129) -> (71.673, 27.2351) centre (71.673, 27.324) ccw
  line L6143 (80.056, 35.418) -> (80.856, 35.418)
  line L6144 (80.056, 35.418) -> (80.856, 35.418)
  arc A4171 (80.473, 28.0351) -> (80.473, 28.2129) centre (80.473, 28.124) ccw
  arc A4172 (71.673, 27.2351) -> (71.673, 27.4129) centre (71.673, 27.324) ccw
  arc A4173 (71.673, 27.4129) -> (71.673, 27.2351) centre (71.673, 27.324) ccw
  arc A4174 (78.397, 37.3974) -> (78.397, 37.0726) centre (78.397, 37.235) ccw
  line L6145 (75.227, 36.068) -> (76.027, 36.068)
  line L6146 (78.656, 36.718) -> (79.456, 36.718)
  line L6147 (77.127, 35.068) -> (77.127, 37.068)
  line L6148 (77.127, 37.068) -> (75.527, 37.068)
  line L6149 (78.656, 36.718) -> (79.456, 36.718)
  arc A4175 (71.673, 27.2351) -> (71.673, 27.4129) centre (71.673, 27.324) ccw
  arc A4176 (72.473, 27.2351) -> (72.473, 27.4129) centre (72.473, 27.324) ccw
  arc A4177 (74.073, 27.2351) -> (74.073, 27.4129) centre (74.073, 27.324) ccw
  arc A4178 (74.073, 27.2351) -> (74.073, 27.4129) centre (74.073, 27.324) ccw
  arc A4179 (72.473, 27.4129) -> (72.473, 27.2351) centre (72.473, 27.324) ccw
  arc A4180 (80.473, 28.2129) -> (80.473, 28.0351) centre (80.473, 28.124) ccw
  line L6150 (48.395, 52.0775) -> (48.395, 54.3505)
  arc A4181 (74.873, 27.2351) -> (74.873, 27.4129) centre (74.873, 27.324) ccw
  arc A4182 (74.073, 27.4129) -> (74.073, 27.2351) centre (74.073, 27.324) ccw
  arc A4183 (74.873, 27.2351) -> (74.873, 27.4129) centre (74.873, 27.324) ccw
  arc A4184 (78.397, 37.0726) -> (78.397, 37.3974) centre (78.397, 37.235) ccw
  arc A4185 (73.273, 27.2351) -> (73.273, 27.4129) centre (73.273, 27.324) ccw
  line L6151 (80.056, 35.418) -> (80.856, 35.418)
  line L6152 (75.227, 36.068) -> (76.027, 36.068)
  arc A4186 (74.873, 27.4129) -> (74.873, 27.2351) centre (74.873, 27.324) ccw
  line L6153 (75.527, 37.068) -> (75.527, 35.068)
  line L6154 (80.056, 36.068) -> (80.856, 36.068)
  line L6155 (78.656, 35.418) -> (79.456, 35.418)
  line L6156 (78.656, 36.068) -> (79.456, 36.068)
  line L6157 (78.656, 36.068) -> (79.456, 36.068)
  arc A4187 (74.968, 37.3974) -> (74.968, 37.0726) centre (74.968, 37.235) ccw
  arc A4188 (74.073, 27.2351) -> (74.073, 27.4129) centre (74.073, 27.324) ccw
  arc A4189 (74.873, 27.4129) -> (74.873, 27.2351) centre (74.873, 27.324) ccw
  arc A4190 (72.473, 27.2351) -> (72.473, 27.4129) centre (72.473, 27.324) ccw
  arc A4191 (80.473, 28.2129) -> (80.473, 28.0351) centre (80.473, 28.124) ccw
  arc A4192 (73.273, 27.4129) -> (73.273, 27.2351) centre (73.273, 27.324) ccw
  arc A4193 (74.873, 27.4129) -> (74.873, 27.2351) centre (74.873, 27.324) ccw
  arc A4194 (73.273, 27.4129) -> (73.273, 27.2351) centre (73.273, 27.324) ccw
  arc A4195 (80.473, 28.0351) -> (80.473, 28.2129) centre (80.473, 28.124) ccw
  arc A4196 (72.473, 27.4129) -> (72.473, 27.2351) centre (72.473, 27.324) ccw
  arc A4197 (73.273, 27.2351) -> (73.273, 27.4129) centre (73.273, 27.324) ccw
  arc A4198 (72.473, 27.4129) -> (72.473, 27.2351) centre (72.473, 27.324) ccw
  arc A4199 (71.673, 27.2351) -> (71.673, 27.4129) centre (71.673, 27.324) ccw
  arc A4200 (74.073, 27.4129) -> (74.073, 27.2351) centre (74.073, 27.324) ccw
  arc A4201 (71.673, 27.4129) -> (71.673, 27.2351) centre (71.673, 27.324) ccw
  arc A4202 (72.473, 27.2351) -> (72.473, 27.4129) centre (72.473, 27.324) ccw
  line L6158 (80.556, 37.068) -> (78.956, 37.068)
  line L6159 (78.956, 37.068) -> (78.956, 35.068)
  arc A4203 (74.873, 27.2351) -> (74.873, 27.4129) centre (74.873, 27.324) ccw
  line L6160 (80.556, 35.068) -> (80.556, 37.068)
  line L6161 (75.227, 36.718) -> (76.027, 36.718)
  line L6162 (75.227, 36.718) -> (76.027, 36.718)
  line L6163 (78.656, 35.418) -> (79.456, 35.418)
  line L6164 (78.656, 36.718) -> (79.456, 36.718)
  line L6165 (80.056, 36.068) -> (80.856, 36.068)
  line L6166 (80.056, 36.718) -> (80.856, 36.718)
  arc A4204 (74.968, 37.0726) -> (74.968, 37.3974) centre (74.968, 37.235) ccw
  line L6167 (80.056, 36.718) -> (80.856, 36.718)
  line L6168 (78.956, 35.068) -> (80.556, 35.068)
  line L6169 (80.056, 36.068) -> (80.856, 36.068)
  line L6170 (77.3, 18.176) -> (76.5, 18.176)
  line L6171 (80.091, 17.272) -> (79.291, 17.272)
  line L6172 (77.3, 17.526) -> (76.5, 17.526)
  line L6173 (77, 16.526) -> (77, 18.526)
  line L6174 (76.627, 36.718) -> (77.427, 36.718)
  line L6175 (76.627, 36.068) -> (77.427, 36.068)
  line L6176 (77.3, 18.176) -> (76.5, 18.176)
  line L6177 (81.191, 16.272) -> (81.191, 18.272)
  line L6178 (80.091, 16.622) -> (79.291, 16.622)
  line L6179 (80.091, 17.922) -> (79.291, 17.922)
  line L6180 (75.4, 18.526) -> (75.4, 16.526)
  line L6181 (77, 18.526) -> (75.4, 18.526)
  line L6182 (78.656, 36.068) -> (79.456, 36.068)
  line L6183 (76.627, 35.418) -> (77.427, 35.418)
  line L6184 (76.627, 35.418) -> (77.427, 35.418)
  line L6185 (76.627, 36.068) -> (77.427, 36.068)
  line L6186 (77.3, 17.526) -> (76.5, 17.526)
  line L6187 (81.491, 16.622) -> (80.691, 16.622)
  line L6188 (81.491, 16.622) -> (80.691, 16.622)
  line L6189 (75.9, 18.176) -> (75.1, 18.176)
  line L6190 (77.3, 18.176) -> (76.5, 18.176)
  line L6191 (75.9, 18.176) -> (75.1, 18.176)
  line L6192 (75.9, 17.526) -> (75.1, 17.526)
  line L6193 (77.3, 17.526) -> (76.5, 17.526)
  line L6194 (80.091, 17.272) -> (79.291, 17.272)
  line L6195 (76.627, 36.718) -> (77.427, 36.718)
  arc A4205 (77.559, 16.1966) -> (77.559, 16.5214) centre (77.559, 16.359) ccw
  line L6196 (77.3, 16.876) -> (76.5, 16.876)
  line L6197 (75.527, 35.068) -> (77.127, 35.068)
  line L6198 (75.227, 35.418) -> (76.027, 35.418)
  line L6199 (75.9, 17.526) -> (75.1, 17.526)
  arc A4206 (81.75, 16.2674) -> (81.75, 15.9426) centre (81.75, 16.105) ccw
  arc A4207 (81.75, 15.9426) -> (81.75, 16.2674) centre (81.75, 16.105) ccw
  line L6200 (79.591, 16.272) -> (81.191, 16.272)
  line L6201 (81.491, 17.272) -> (80.691, 17.272)
  line L6202 (81.491, 17.922) -> (80.691, 17.922)
  line L6203 (80.056, 36.718) -> (80.856, 36.718)
  line L6204 (81.491, 16.622) -> (80.691, 16.622)
  line L6205 (81.191, 18.272) -> (79.591, 18.272)
  line L6206 (80.091, 17.922) -> (79.291, 17.922)
  line L6207 (76.627, 36.068) -> (77.427, 36.068)
  line L6208 (75.227, 35.418) -> (76.027, 35.418)
  line L6209 (79.591, 18.272) -> (79.591, 16.272)
  line L6210 (75.227, 35.418) -> (76.027, 35.418)
  line L6211 (81.491, 17.272) -> (80.691, 17.272)
  line L6212 (81.491, 17.922) -> (80.691, 17.922)
  line L6213 (81.491, 17.272) -> (80.691, 17.272)
  line L6214 (75.227, 36.068) -> (76.027, 36.068)
  line L6215 (80.091, 17.922) -> (79.291, 17.922)
  line L6216 (76.627, 36.718) -> (77.427, 36.718)
  line L6217 (76.627, 35.418) -> (77.427, 35.418)
  line L6218 (81.491, 17.922) -> (80.691, 17.922)
  line L6219 (77.0382, 47.498) -> (77.6478, 47.498)
  line L6220 (77.0382, 46.482) -> (77.0382, 47.498)
  line L6221 (83.693, 27.145) -> (83.693, 26.795)
  arc A4208 (83.543, 27.1132) -> (83.543, 27.1767) centre (83.543, 27.145) ccw
  line L6222 (78.786, 47.54) -> (78.186, 47.54)
  arc A4209 (69.192, 22.6682) -> (69.192, 22.7317) centre (69.192, 22.7) ccw
  line L6223 (69.1642, 21.8948) -> (69.5198, 21.8948)
  line L6224 (78.7908, 46.865) -> (78.7908, 47.115)
  line L6225 (78.7908, 47.498) -> (78.7908, 46.482)
  line L6226 (78.1812, 46.482) -> (78.1812, 47.498)
  arc A4210 (69.192, 21.7818) -> (69.192, 21.7183) centre (69.192, 21.75) ccw
  arc A4211 (69.492, 21.7818) -> (69.492, 21.7183) centre (69.492, 21.75) ccw
  line L6227 (78.7908, 46.482) -> (78.1812, 46.482)
  line L6228 (78.186, 47.54) -> (78.186, 46.44)
  line L6229 (69.1642, 22.5552) -> (69.1642, 21.8948)
  line L6230 (78.7908, 47.498) -> (78.7908, 46.482)
  line L6231 (78.1812, 46.482) -> (78.1812, 47.498)
  line L6232 (72.261, 57.3278) -> (72.011, 57.3278)
  line L6233 (78.1812, 46.865) -> (78.7908, 46.865)
  line L6234 (69.342, 21.75) -> (69.342, 22.1)
  arc A4212 (69.492, 22.7317) -> (69.492, 22.6682) centre (69.492, 22.7) ccw
  line L6235 (69.342, 22.35) -> (69.342, 22.7)
  line L6236 (69.492, 21.75) -> (69.492, 22.7)
  line L6237 (69.5198, 22.5552) -> (69.1642, 22.5552)
  line L6238 (69.1642, 21.8948) -> (69.5198, 21.8948)
  line L6239 (78.186, 46.44) -> (78.786, 46.44)
  arc A4213 (69.192, 21.7183) -> (69.192, 21.7818) centre (69.192, 21.75) ccw
  line L6240 (69.342, 21.75) -> (69.342, 22.1)
  line L6241 (69.342, 22.35) -> (69.342, 22.7)
  line L6242 (69.177, 22.54) -> (69.177, 21.91)
  line L6243 (69.5198, 21.8948) -> (69.5198, 22.5552)
  line L6244 (69.507, 22.54) -> (69.177, 22.54)
  line L6245 (69.492, 22.7) -> (69.192, 22.7)
  line L6246 (78.1812, 47.498) -> (78.7908, 47.498)
  line L6247 (69.507, 21.91) -> (69.507, 22.54)
  line L6248 (78.7908, 47.115) -> (78.1812, 47.115)
  line L6249 (69.342, 22.35) -> (69.342, 22.7)
  arc A4214 (69.492, 22.6682) -> (69.492, 22.7317) centre (69.492, 22.7) ccw
  line L6250 (69.192, 21.75) -> (69.492, 21.75)
  line L6251 (78.1812, 47.498) -> (78.7908, 47.498)
  line L6252 (78.7908, 46.482) -> (78.1812, 46.482)
  line L6253 (69.5198, 21.8948) -> (69.5198, 22.5552)
  line L6254 (78.1812, 47.115) -> (78.1812, 46.865)
  line L6255 (69.342, 21.75) -> (69.342, 22.1)
  line L6256 (76.583, 52.2478) -> (76.583, 51.6382)
  line L6257 (83.858, 26.985) -> (83.528, 26.985)
  line L6258 (77.6478, 46.482) -> (77.0382, 46.482)
  line L6259 (77.043, 46.44) -> (77.643, 46.44)
  line L6260 (77.643, 46.44) -> (77.643, 47.54)
  line L6261 (77.643, 47.54) -> (77.043, 47.54)
  arc A4215 (83.543, 26.2268) -> (83.543, 26.1633) centre (83.543, 26.195) ccw
  line L6262 (83.693, 26.545) -> (83.693, 26.195)
  line L6263 (77.6478, 47.498) -> (77.6478, 46.482)
  arc A4216 (83.543, 27.1767) -> (83.543, 27.1132) centre (83.543, 27.145) ccw
  line L6264 (83.5152, 27.0002) -> (83.5152, 26.3398)
  line L6265 (76.158, 51.643) -> (77.258, 51.643)
  line L6266 (77.6478, 46.865) -> (77.6478, 47.115)
  line L6267 (77.0382, 47.498) -> (77.6478, 47.498)
  line L6268 (83.693, 27.145) -> (83.693, 26.795)
  line L6269 (15.746, 24.6888) -> (15.496, 24.6888)
  line L6270 (73.406, 53.5178) -> (74.422, 53.5178)
  line L6271 (73.364, 53.513) -> (73.364, 52.913)
  line L6272 (72.2122, 54.229) -> (72.2122, 55.245)
  line L6273 (72.217, 55.287) -> (72.217, 54.187)
  line L6274 (72.8218, 54.862) -> (72.2122, 54.862)
  line L6275 (15.496, 24.6888) -> (15.496, 24.0792)
  line L6276 (73.789, 53.5178) -> (73.789, 52.9082)
  line L6277 (15.496, 24.0792) -> (15.746, 24.0792)
  line L6278 (72.217, 54.187) -> (72.817, 54.187)
  line L6279 (72.8218, 55.245) -> (72.8218, 54.229)
  line L6280 (74.422, 53.5178) -> (74.422, 52.9082)
  line L6281 (72.2122, 55.245) -> (72.8218, 55.245)
  line L6282 (72.2122, 54.229) -> (72.2122, 55.245)
  line L6283 (73.406, 52.9082) -> (73.406, 53.5178)
  line L6284 (74.464, 53.513) -> (73.364, 53.513)
  line L6285 (73.406, 53.5178) -> (74.422, 53.5178)
  line L6286 (74.039, 53.5178) -> (73.789, 53.5178)
  line L6287 (74.464, 52.913) -> (74.464, 53.513)
  line L6288 (72.644, 56.7182) -> (71.628, 56.7182)
  line L6289 (71.586, 56.723) -> (72.686, 56.723)
  line L6290 (73.789, 52.9082) -> (74.039, 52.9082)
  line L6291 (72.686, 56.723) -> (72.686, 57.323)
  line L6292 (73.364, 52.913) -> (74.464, 52.913)
  line L6293 (72.686, 57.323) -> (71.586, 57.323)
  line L6294 (72.8218, 54.229) -> (72.2122, 54.229)
  line L6295 (72.817, 55.287) -> (72.217, 55.287)
  line L6296 (74.422, 53.5178) -> (74.422, 52.9082)
  line L6297 (72.8218, 54.229) -> (72.2122, 54.229)
  line L6298 (72.8218, 55.245) -> (72.8218, 54.229)
  line L6299 (72.2122, 54.612) -> (72.8218, 54.612)
  line L6300 (16.129, 24.6888) -> (16.129, 24.0792)
  line L6301 (71.586, 57.323) -> (71.586, 56.723)
  line L6302 (72.8218, 54.612) -> (72.8218, 54.862)
  line L6303 (74.039, 52.9082) -> (74.039, 53.5178)
  line L6304 (72.644, 57.3278) -> (72.644, 56.7182)
  line L6305 (72.011, 57.3278) -> (72.011, 56.7182)
  line L6306 (71.628, 56.7182) -> (71.628, 57.3278)
  line L6307 (71.628, 56.7182) -> (71.628, 57.3278)
  line L6308 (72.644, 56.7182) -> (71.628, 56.7182)
  line L6309 (74.422, 52.9082) -> (73.406, 52.9082)
  line L6310 (72.644, 57.3278) -> (72.644, 56.7182)
  line L6311 (71.628, 57.3278) -> (72.644, 57.3278)
  line L6312 (72.2122, 55.245) -> (72.8218, 55.245)
  line L6313 (72.817, 54.187) -> (72.817, 55.287)
  line L6314 (72.2122, 54.862) -> (72.2122, 54.612)
  line L6315 (71.628, 57.3278) -> (72.644, 57.3278)
  line L6316 (73.406, 52.9082) -> (73.406, 53.5178)
  line L6317 (69.5198, 22.5552) -> (69.1642, 22.5552)
  line L6318 (16.129, 24.0792) -> (15.113, 24.0792)
  line L6319 (74.422, 52.9082) -> (73.406, 52.9082)
  line L6320 (72.011, 56.7182) -> (72.261, 56.7182)
  line L6321 (15.73, 19.8688) -> (15.73, 19.2592)
  line L6322 (18.969, 26.331) -> (18.369, 26.331)
  line L6323 (18.9738, 26.289) -> (18.9738, 25.273)
  line L6324 (18.9738, 25.273) -> (18.3642, 25.273)
  line L6325 (18.369, 25.231) -> (18.969, 25.231)
  line L6326 (24.4168, 11.565) -> (24.4168, 11.815)
  line L6327 (24.4168, 11.182) -> (23.8072, 11.182)
  line L6328 (18.3642, 25.656) -> (18.9738, 25.656)
  line L6329 (14.672, 19.864) -> (14.672, 19.264)
  line L6330 (18.3642, 25.273) -> (18.3642, 26.289)
  line L6331 (15.071, 24.684) -> (15.071, 24.084)
  line L6332 (18.9738, 25.906) -> (18.3642, 25.906)
  line L6333 (16.129, 24.6888) -> (16.129, 24.0792)
  line L6334 (18.3642, 26.289) -> (18.9738, 26.289)
  line L6335 (15.071, 24.084) -> (16.171, 24.084)
  line L6336 (14.714, 19.2592) -> (14.714, 19.8688)
  line L6337 (14.714, 19.8688) -> (15.73, 19.8688)
  line L6338 (72.261, 56.7182) -> (72.261, 57.3278)
  line L6339 (16.171, 24.684) -> (15.071, 24.684)
  arc A4217 (83.543, 26.1633) -> (83.543, 26.2268) centre (83.543, 26.195) ccw
  line L6340 (83.528, 26.355) -> (83.858, 26.355)
  line L6341 (77.6478, 46.482) -> (77.0382, 46.482)
  line L6342 (83.858, 26.355) -> (83.858, 26.985)
  line L6343 (83.528, 26.985) -> (83.528, 26.355)
  line L6344 (83.5152, 26.3398) -> (83.8708, 26.3398)
  arc A4218 (69.192, 22.7317) -> (69.192, 22.6682) centre (69.192, 22.7) ccw
  line L6345 (77.6478, 47.115) -> (77.0382, 47.115)
  line L6346 (69.1642, 22.5552) -> (69.1642, 21.8948)
  line L6347 (83.693, 27.145) -> (83.693, 26.795)
  line L6348 (83.8708, 27.0002) -> (83.5152, 27.0002)
  line L6349 (78.786, 46.44) -> (78.786, 47.54)
  line L6350 (69.192, 22.7) -> (69.192, 21.75)
  line L6351 (69.177, 21.91) -> (69.507, 21.91)
  arc A4219 (69.492, 21.7183) -> (69.492, 21.7818) centre (69.492, 21.75) ccw
  line L6352 (23.8072, 11.182) -> (23.8072, 12.198)
  line L6353 (18.3642, 25.273) -> (18.3642, 26.289)
  line L6354 (18.369, 26.331) -> (18.369, 25.231)
  line L6355 (15.772, 19.264) -> (15.772, 19.864)
  line L6356 (23.8072, 11.815) -> (23.8072, 11.565)
  line L6357 (15.369, 18.0848) -> (15.369, 17.4752)
  line L6358 (14.944, 16.937) -> (14.944, 16.337)
  line L6359 (14.944, 17.48) -> (16.044, 17.48)
  line L6360 (55.2958, 56.898) -> (55.2958, 57.148)
  line L6361 (24.412, 12.24) -> (23.812, 12.24)
  line L6362 (83.82, 28.2448) -> (83.82, 27.6352)
  line L6363 (83.82, 27.6352) -> (82.804, 27.6352)
  line L6364 (20.909, 11.007) -> (21.509, 11.007)
  line L6365 (16.044, 17.48) -> (16.044, 18.08)
  line L6366 (82.804, 27.6352) -> (82.804, 28.2448)
  line L6367 (23.812, 11.14) -> (24.412, 11.14)
  line L6368 (23.812, 12.24) -> (23.812, 11.14)
  line L6369 (23.8072, 11.565) -> (24.4168, 11.565)
  line L6370 (21.509, 11.007) -> (21.509, 12.107)
  line L6371 (20.9042, 12.065) -> (21.5138, 12.065)
  line L6372 (82.762, 28.24) -> (82.762, 27.64)
  line L6373 (55.2958, 57.148) -> (54.6862, 57.148)
  line L6374 (15.619, 18.0848) -> (15.369, 18.0848)
  line L6375 (15.619, 17.4752) -> (15.619, 18.0848)
  line L6376 (82.804, 27.6352) -> (82.804, 28.2448)